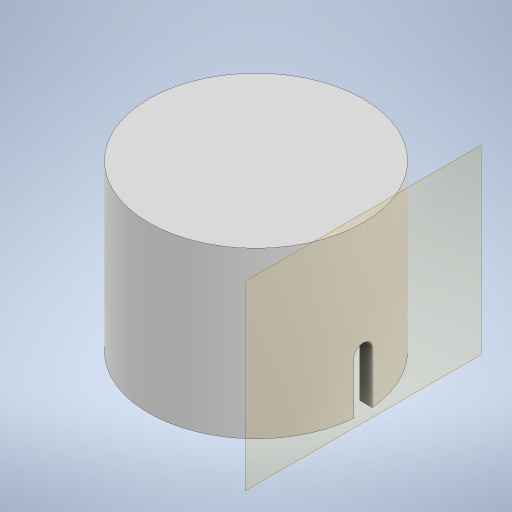
# Autodesk Inventor part: TopPotentiometer
Saved by Autodesk Inventor 2024 (Build 280153000, 153)
## iProperties
Created: 2023-10-09
Part Number: TopPotentiometer
Material: Generic
Document SubType Name: Modeling
Designer: Gibi500
Density: 1 g/cm^3
Appearance: Default
Author: Gibi500
## iProperties of the stored document TopPotentiometer_3DPrint.ipt
Created: 2023-10-09
Part Number: TopPotentiometer_3DPrint
Material: Generic
Document SubType Name: Modeling
Designer: Gibi500
Density: 1 g/cm^3
Appearance: Default
Author: Gibi500
Autodesk Inventor part; units mm, degrees
ref_plane "XZ Plane" through (0, 0, 0) normal (0, 1, 0) x (-1, 0, 0)
ref_plane "XY Plane" through (0, 0, 0) normal (0, 0, 1) x (1, 0, 0)
sketch "Sketch1" plane through (0, 0, 0) normal (0, 1, 0) x (-1, 0, 0)
  circle A0 centre (0, 0) radius 23
  circle A1 centre (0, 0) radius 26
  dimension "d0" = 46
  dimension "d1" = 52
  constraints: 2 centre point, 2 coincident
  measures "d0" diameter of A0
  measures "d1" diameter of A1
extrude "Extrusion1" add sketch "Sketch1" along normal blind 35
sketch "Sketch2" plane through (0, 35, 0) normal (0, 1, 0) x (1, 0, 0)
  circle A0 centre (0, 0) radius 26
  constraints: 1 centre point, 1 coincident
extrude "Extrusion2" add sketch "Sketch2" along normal blind 5
sketch "Sketch3" plane through (0, 35, 0) normal (0, -1, 0) x (1, 0, 0)
  line L0 (-12.7, 12.7) -> (12.7, 12.7)
  line L1 (12.7, 12.7) -> (12.7, -12.7)
  line L2 (12.7, -12.7) -> (-12.7, -12.7)
  line L3 (-12.7, -12.7) -> (-12.7, 12.7)
  line L4 (-12.7, 12.7) -> (12.7, -12.7) construction
  line L5 (12.7, 12.7) -> (-12.7, -12.7) construction
  circle A0 centre (12.7, 12.7) radius 2.5
  circle A1 centre (12.7, -12.7) radius 2.5
  circle A2 centre (-12.7, -12.7) radius 2.5
  circle A3 centre (-12.7, 12.7) radius 2.5
  circle A4 centre (12.7, 12.7) radius 1
  circle A5 centre (12.7, -12.7) radius 1
  circle A6 centre (-12.7, -12.7) radius 1
  circle A7 centre (-12.7, 12.7) radius 1
  point P0 (0, 0)
  dimension "d6" = 25.4
  dimension "d7" = 25.4
  dimension "d8" = 5
  dimension "d9" = 5
  dimension "d10" = 5
  dimension "d11" = 5
  dimension "d14" = 2
  dimension "d15" = 2
  dimension "d16" = 2
  dimension "d17" = 2
  constraints: 12 end point, 8 centre point, 8 coincident, 2 midpoint, 2 parallel, 1 horizontal, 1 perpendicular
  measures "d6" distance of L1.end L2.end
  measures "d7" distance of L0.end L1.end
  measures "d8" diameter of A0
  measures "d9" diameter of A1
  measures "d10" diameter of A2
  measures "d11" diameter of A3
  measures "d14" diameter of A4
  measures "d15" diameter of A5
  measures "d16" diameter of A6
  measures "d17" diameter of A7
extrude "Extrusion3" add sketch "Sketch3" along normal blind 5 contours A7 L3 A3 L0 | L0 A3 L3 A7 | A0 L1 A4 L0 | L0 A4 L1 A0 | A2 L2 A6 L3 | L3 A6 L2 A2 | A1 L2 A5 L1 | L1 A5 L2 A1
ref_plane "Work Plane1" through (26, 0, 0) normal (1, 0, 0) x (0, 1, 0)
sketch "Sketch4" plane through (26, 0, 0) normal (1, 0, 0) x (0, 1, 0)
  line L0 (0, 0) -> (12.5, 0) construction
  line L1 (0, -2.25) -> (12.5, -2.25)
  line L2 (12.5, 2.25) -> (0, 2.25)
  arc A0 (0, 2.25) -> (0, -2.25) centre (0, 0) ccw
  arc A1 (12.5, -2.25) -> (12.5, 2.25) centre (12.5, 0) ccw
  point P0 (0, 0)
  point P1 (6.25, 0)
  dimension "d19" = 12.5
  dimension "d20" = 4.5
  constraints: 8 end point, 4 point on circle, 4 tangent, 2 centre point, 1 coincident, 1 horizontal, 1 midpoint, 1 parallel
  measures "d19" distance of L0.start L0.end
  measures "d20" diameter of A1
extrude "Extrusion4" cut sketch "Sketch4" against normal through all
body "Solid1"
